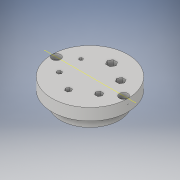
# Autodesk Inventor part: AllenKeyHolder
Saved by Autodesk Inventor 2019.1 (Build 231200000, 200)
## iProperties
Created: 2018-08-31
Part Number: AllenKeyHolder
Material: Generic
Document SubType Name: Modeling
Designer: steele
Density: 1 g/cm^3
Appearance: Default
Author: steele
Autodesk Inventor part; units mm, degrees
ref_plane "YZ Plane" through (0, 0, 0) normal (1, 0, 0) x (0, 1, 0)
ref_plane "XZ Plane" through (0, 0, 0) normal (0, 1, 0) x (-1, 0, 0)
ref_plane "XY Plane" through (0, 0, 0) normal (0, 0, 1) x (1, 0, 0)
sketch "Sketch1" plane through (0, 0, 0) normal (0, 1, 0) x (-1, 0, 0)
  circle A0 centre (0, 0) radius 20.574
  dimension "d0" = 41.148
  constraints: 1 centre point, 1 coincident
  measures "d0" diameter of A0
extrude "Extrusion1" add sketch "Sketch1" against normal blind 6.35
sketch "Sketch2" plane through (0, -6.35, 0) normal (0, -1, 0) x (1, 0, 0)
  circle A0 centre (0, 0) radius 15.875
  dimension "d3" = 31.75
  constraints: 1 centre point, 1 coincident
  measures "d3" diameter of A0
extrude "Extrusion2" add sketch "Sketch2" along normal blind 6.35
sketch "Sketch4" plane through (0, 0, 0) normal (0, 1, 0) x (1, 0, 0)
  circle A0 centre (0, 0) radius 20.574 projected
  point P0 (18.2245, 0)
  point P1 (-18.2245, 0)
  dimension "d9" = 18.2245
  dimension "d10" = 18.2245
  measures "d9" distance of point (18.224, 0) A0.centre
  measures "d10" distance of point (0, 0) point (-18.224, 0)
hole "Hole1" at (18.2245, 0, 0) at (-18.2245, 0, 0) direction (0, -1, 0) diameter 3.2766 end through all counterbore diameter 4.6482 counterbore depth 2.8448 clearance for "Socket Head Cap Screw" size "#4" standard "Ansi Unified Screw Threads"
sketch "Sketch5" plane through (0, 0, 0) normal (0, 1, 0) x (1, 0, 0)
  circle A0 centre (0, 0) radius 12.065 construction
  line L0 (2.055, 12.0593) -> (0.8425, 9.9593)
  line L1 (0.8425, 9.9593) -> (-1.5823, 9.9593)
  line L2 (-1.5823, 9.9593) -> (-2.7948, 12.0593)
  line L3 (-2.7948, 12.0593) -> (-1.5823, 14.1593)
  line L4 (-1.5823, 14.1593) -> (0.8425, 14.1593)
  line L5 (0.8425, 14.1593) -> (2.055, 12.0593)
  line L6 (12.3949, 6.35) -> (11.3268, 4.5)
  line L7 (11.3268, 4.5) -> (9.1906, 4.5)
  line L8 (9.1906, 4.5) -> (8.1225, 6.35)
  line L9 (8.1225, 6.35) -> (9.1906, 8.2)
  line L10 (9.1906, 8.2) -> (11.3268, 8.2)
  line L11 (11.3268, 8.2) -> (12.3949, 6.35)
  line L12 (-28.8036, 0) -> (28.8036, 0) projected
  line L13 (11.5524, -4.1093) -> (12.4762, -5.7093)
  line L14 (12.4762, -5.7093) -> (11.5524, -7.3093)
  line L15 (11.5524, -7.3093) -> (9.7049, -7.3093)
  line L16 (9.7049, -7.3093) -> (8.7811, -5.7093)
  line L17 (8.7811, -5.7093) -> (9.7049, -4.1093)
  line L18 (9.7049, -4.1093) -> (11.5524, -4.1093)
  line L19 (1.1493, -10.7093) -> (1.9287, -12.0593)
  line L20 (1.9287, -12.0593) -> (1.1493, -13.4093)
  line L21 (1.1493, -13.4093) -> (-0.4095, -13.4093)
  line L22 (-0.4095, -13.4093) -> (-1.189, -12.0593)
  line L23 (-1.189, -12.0593) -> (-0.4095, -10.7093)
  line L24 (-0.4095, -10.7093) -> (1.1493, -10.7093)
  line L25 (-8.9886, -6.35) -> (-9.6237, -7.45)
  line L26 (-9.6237, -7.45) -> (-10.8938, -7.45)
  line L27 (-10.8938, -7.45) -> (-11.5289, -6.35)
  line L28 (-11.5289, -6.35) -> (-10.8938, -5.25)
  line L29 (-10.8938, -5.25) -> (-9.6237, -5.25)
  line L30 (-9.6237, -5.25) -> (-8.9886, -6.35)
  line L31 (-9.6471, 5.7093) -> (-10.1379, 4.8593)
  line L32 (-10.1379, 4.8593) -> (-11.1194, 4.8593)
  line L33 (-11.1194, 4.8593) -> (-11.6101, 5.7093)
  line L34 (-11.6101, 5.7093) -> (-11.1194, 6.5593)
  line L35 (-11.1194, 6.5593) -> (-10.1379, 6.5593)
  line L36 (-10.1379, 6.5593) -> (-9.6471, 5.7093)
  point P0 (-0.3699, 12.0593)
  point P1 (-10.6286, 5.7093)
  point P2 (-10.2587, -6.35)
  point P3 (0.3699, -12.0593)
  point P4 (10.6286, -5.7093)
  point P5 (10.2587, 6.35)
  point P6 (-0.3699, 12.0593)
  point P7 (10.2587, 6.35)
  point P8 (10.6286, -5.7093)
  point P9 (0.3699, -12.0593)
  point P10 (-10.2587, -6.35)
  point P11 (-10.6286, 5.7093)
  dimension "d18" = 24.13
  dimension "d21" = 360
  dimension "d23" = 4.2
  dimension "d24" = 3.7
  dimension "d25" = 3.2
  dimension "d26" = 2.7
  dimension "d27" = 2.2
  dimension "d28" = 1.7
  constraints: 72 end point, 7 coincident, 5 parallel, 88 other
  measures "d23" distance between parallel lines of L1 L4
  measures "d24" distance between parallel lines of L7 L10
  measures "d25" distance between parallel lines of L15 L18
  measures "d26" distance between parallel lines of L21 L24
  measures "d27" distance between parallel lines of L26 L29
  measures "d28" distance between parallel lines of L32 L35
extrude "Extrusion4" cut sketch "Sketch5" against normal through all
equation "\"d0\" = outerDiameter"
equation "\"d3\" = innerDiameter"
equation "\"d9\" = screwRadius"
equation "\"d10\" = screwRadius"
equation "\"d23\" = allenKeyHole4_0mm"
equation "\"d24\" = allenKeyHole3_5mm"
equation "\"d25\" = allenKeyHole3_0mm"
equation "\"d26\" = allenKeyHole2_5mm"
equation "\"d27\" = allenKeyHole2_0mm"
equation "\"d28\" = allenKeyHold1_5mm"
equation "\"innerDiameter\" = 31.75"
equation "\"edgeRadius\" = 4.699"
equation "\"allenKey3_0mm\" = 3"
equation "\"allenKeyClearance\" = 0.2"
equation "\"allenKeyHole3_0mm\" = allenKey3_0mm + allenKeyClearance"
equation "\"screwRadius\" = 0.5 * innerDiameter + 0.5 * edgeRadius"
equation "\"allenKey4_0mm\" = 4"
equation "\"allenKey3_5mm\" = 3.5"
equation "\"allenKey2_5mm\" = 2.5"
equation "\"alleyKey2_0mm\" = 2"
equation "\"allenKey1_5mm\" = 1.5"
equation "\"allenKeyHole4_0mm\" = allenKey4_0mm + allenKeyClearance"
equation "\"allenKeyHole2_5mm\" = allenKey2_5mm + allenKeyClearance"
equation "\"allenKeyHole2_0mm\" = alleyKey2_0mm + allenKeyClearance"
equation "\"allenKeyHole3_5mm\" = allenKey3_5mm + allenKeyClearance"
equation "\"allenKeyHold1_5mm\" = allenKey1_5mm + allenKeyClearance"
equation "\"outerDiameter\" = 41.148"
body "Solid1"
